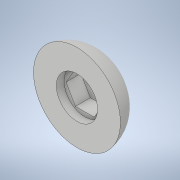
# Autodesk Inventor part: nut_cover1
Saved by Autodesk Inventor 2020 (Build 240168000, 168)
## iProperties
Created: 2018-05-22
Part Number: nut_cover1
Material: Generic
Document SubType Name: Modeling
Designer: stedrock
Density: 1 g/cm^3
Appearance: Default
Author: stedrock
Autodesk Inventor part; units mm, degrees
ref_plane "YZ Plane" through (0, 0, 0) normal (1, 0, 0) x (0, 1, 0)
ref_plane "XZ Plane" through (0, 0, 0) normal (0, 1, 0) x (-1, 0, 0)
ref_plane "XY Plane" through (0, 0, 0) normal (0, 0, 1) x (1, 0, 0)
sketch "Sketch1" plane through (0, 0, 0) normal (0, 0, 1) x (1, 0, 0)
  line L0 (0, 0) -> (26.2535, 0) construction
  line L1 (4.3301, 0) -> (2.1651, -3.75)
  line L2 (2.1651, -3.75) -> (-2.1651, -3.75)
  line L3 (-2.1651, -3.75) -> (-4.3301, 0)
  line L4 (-4.3301, 0) -> (-2.1651, 3.75)
  line L5 (-2.1651, 3.75) -> (2.1651, 3.75)
  line L6 (2.1651, 3.75) -> (4.3301, 0)
  circle A0 centre (0, 0) radius 4.75
  circle A1 centre (0, 0) radius 5.75
  dimension "d0" = 7.5
  dimension "d1" = 9.5
  dimension "d2" = 11.5
  constraints: 14 end point, 3 coincident, 2 centre point, 1 horizontal, 1 point on line, 13 other
  measures "d0" distance between parallel lines of L1 L4
  measures "d1" diameter of A0
  measures "d2" diameter of A1
sketch "Sketch3" plane through (0, 0, 0) normal (0, 1, 0) x (-1, 0, 0)
  line L0 (0, 0) -> (0, -4.2)
  line L1 (5.75, 0) -> (-5.75, 0) projected
  line L2 (0, 0) -> (-26.2535, 0) construction
  line L3 (-5.75, 0) -> (0, 0)
  line L4 (-5.75, 0) -> (-5.75, 1.8)
  line L5 (0, -4.2) -> (-4.3301, -4.2)
  line L6 (-4.3301, 0) -> (-2.1651, 0) projected
  line L7 (-2.1651, 0) -> (-4.3301, 0) projected
  line L8 (-4.3301, -4.2) -> (-4.3301, 0) construction
  line L9 (4.75, 0) -> (-4.75, 0) projected
  line L10 (-5.75, 0) -> (-4.75, 0)
  line L11 (-4.75, 0) -> (-4.75, 1.8)
  line L12 (-4.75, 1.8) -> (-5.75, 1.8)
  line L13 (-5.75, 1.8) -> (-5.75, 0)
  line L14 (-5.75, 1.8) -> (-10, 1.8)
  arc A0 (-5.9613, -3.8234) -> (-4.3301, -4.2) centre (-4.3301, -0.4792) ccw
  arc A1 (-10, 1.8) -> (-5.9613, -3.8234) centre (-2.7617, 2.7366) ccw
  dimension "d3" = 4.2
  dimension "d9" = 1.8
  dimension "d10" = 10
  constraints: 21 end point, 4 horizontal, 4 point on circle, 3 parallel, 2 centre point, 2 tangent, 2 vertical, 1 perpendicular, 1 other
  measures "d3" distance of L0.start L0.end
  measures "d9" distance of L9.end L11.end
  measures "d10" distance from line of L14.end L0
revolve "Revolution1" add sketch "Sketch3" angle 360 about axis through (0, 0, 0) along (0, 0, -1)
extrude "Extrusion1" cut sketch "Sketch1" against normal blind 3.45 contours L1 L2 L3 L4 L5 L6
body "Solid1"
